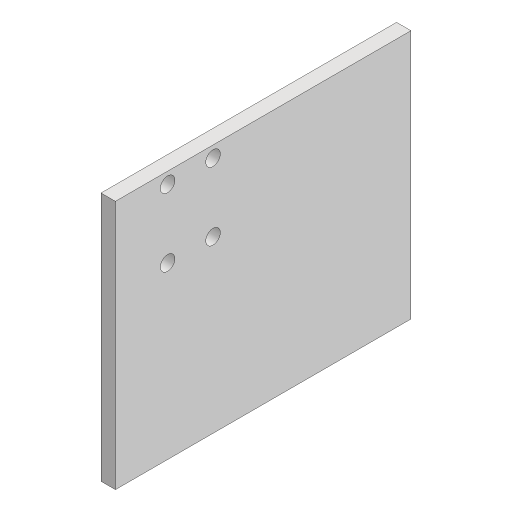
# Autodesk Inventor part: LinearSlidePlate
Saved by Autodesk Inventor 2023 (Build 270158000, 158)
## iProperties
Created: 2022-10-31
Part Number: LinearSlidePlate
Material: Generic
Document SubType Name: Modeling
Designer: deli
Density: 1 g/cm^3
Appearance: Default
Author: deli
Autodesk Inventor part; units mm, degrees
ref_plane "YZ Plane" through (0, 0, 0) normal (1, 0, 0) x (0, 1, 0)
ref_plane "XZ Plane" through (0, 0, 0) normal (0, 1, 0) x (-1, 0, 0)
ref_plane "XY Plane" through (0, 0, 0) normal (0, 0, 1) x (1, 0, 0)
sketch "Sketch1" plane through (0, 0, 0) normal (1, 0, 0) x (0, 1, 0)
  circle A0 centre (15.6311, -24.6287) radius 1.6
  circle A1 centre (15.6311, -34.6287) radius 1.6
  circle A2 centre (0.6311, -24.6287) radius 1.6
  circle A3 centre (0.6311, -34.6287) radius 1.6
  line L0 (15.6311, -24.6287) -> (15.6311, -34.6287) construction
  line L1 (15.6311, -34.6287) -> (0.6311, -34.6287) construction
  line L2 (0.6311, -34.6287) -> (0.6311, -24.6287) construction
  line L3 (0.6311, -24.6287) -> (15.6311, -24.6287) construction
  line L4 (18.1311, -13.1287) -> (-36.8689, -13.1287)
  line L5 (-36.8689, -13.1287) -> (-36.8689, -78.2287)
  line L6 (-36.8689, -78.2287) -> (18.1311, -78.2287)
  line L7 (18.1311, -78.2287) -> (18.1311, -13.1287)
  circle A4 centre (-10.4689, -74.2287) radius 2
  circle A5 centre (-20.4689, -74.2287) radius 2
  circle A6 centre (-10.4689, -24.6287) radius 2
  circle A7 centre (-20.4689, -24.6287) radius 2
  line L8 (-10.4689, -74.2287) -> (-20.4689, -74.2287) construction
  line L9 (-20.4689, -74.2287) -> (-20.4689, -24.6287) construction
  line L10 (-20.4689, -24.6287) -> (-10.4689, -24.6287) construction
  line L11 (-10.4689, -24.6287) -> (-10.4689, -74.2287) construction
  line L12 (-4.9689, -69.9287) -> (-4.9689, -28.9287)
  line L13 (-4.9689, -28.9287) -> (-25.9689, -28.9287)
  line L14 (-25.9689, -28.9287) -> (-25.9689, -69.9287)
  line L15 (-25.9689, -69.9287) -> (-4.9689, -69.9287)
  circle A8 centre (-29.3689, -16.6287) radius 1
  circle A9 centre (-14.3689, -16.6287) radius 1
  circle A10 centre (-3.3873, -16.6287) radius 1
  circle A11 centre (11.2682, -16.6287) radius 1
  point P0 (0, 0)
  dimension "d0" = 3.2
  dimension "d1" = 10
  dimension "d2" = 15
  dimension "d4" = 2.5
  dimension "d9" = 4
  dimension "d10" = 10
  dimension "d11" = 49.6
  dimension "d12" = 21
  dimension "d13" = 41
  dimension "d14" = 5.5
  dimension "d15" = 4.3
  dimension "d18" = 11.5
  dimension "d19" = 55
  dimension "d21" = 2
  dimension "d23" = 3.5
  dimension "d24" = 3.5
  dimension "d25" = 15
  dimension "d26" = 7.5
  dimension "d27" = 3.5
  dimension "d28" = 3.5
  dimension "d29" = 4
  dimension "d31" = 2
  constraints: 32 end point, 12 centre point, 9 equal radius, 8 perpendicular, 5 parallel, 1 collinear, 1 horizontal, 1 vertical
  measures "d0" diameter of A0
  measures "d1" distance of L0.start L0.end
  measures "d2" distance of L2.end L0.start
  measures "d4" distance from line of L7 L0.start
  measures "d9" diameter of A4
  measures "d10" distance of L8.start L8.end
  measures "d11" distance of L10.end L8.start
  measures "d12" distance of L14.end L12.start
  measures "d13" distance of L12.start L12.end
  measures "d14" distance between parallel lines of L11 L12
  measures "d15" distance between parallel lines of L8 L15
  measures "d18" distance from line of L2.end L4
  measures "d19" distance of L4.start L4.end
  measures "d21" diameter of A8
  measures "d23" distance from line of L4 A8.centre
  measures "d24" distance from line of L4 A9.centre
  measures "d25" distance of A8.centre A9.centre
  measures "d26" distance from line of L5 A8.centre
  measures "d27" distance from line of L4 A10.centre
  measures "d28" distance from line of L4 A11.centre
  measures "d29" distance edge to line of A3 L12
  measures "d31" distance edge to line of A4 L6
extrude "Extrusion1" add sketch "Sketch1" along normal blind 3.175 contours L7 L6 L5 L4 | A4 | A5 | A6 | A7 | L15 L14 L13 L12 | A8 | A9 | A10 | A11
equation "\"d14\" = -0.5 * d10 + 0.5 * d12"
equation "\"d15\" = -0.5 * d13 + 0.5 * d11"
equation "\"d27\" = d24"
equation "\"d28\" = d23"
body "Solid1"
